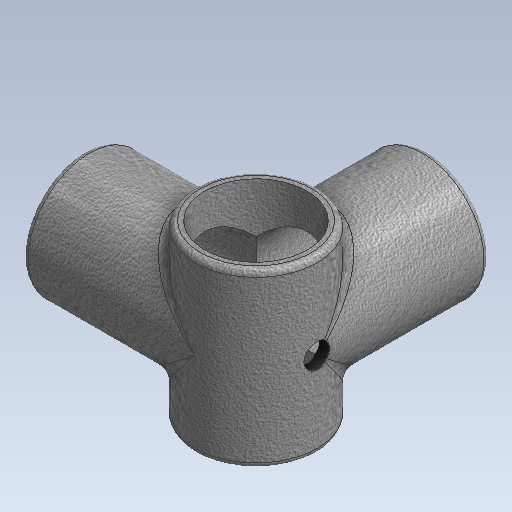
# Autodesk Inventor part: L21-6
Saved by Autodesk Inventor 2021 (Build 250183000, 183)
## iProperties
Created: 2020-04-23
Part Number: L21-6
Material: Aluminium Cast
Document SubType Name: Modeling
Designer: Hannah
Density: 3.00366 g/cm^3
Appearance: Aluminum Cast
Mass: 160 g
Surface Area: 314.88 cm^2
Volume: 53.2684 cm^3
Vendor: Kee Systems
Description: 90 deg side outlet tee
Catalog Web Link: https://keesystems.com/store/fittings/kee-lite/l21-side-outlet-tee.html
Size: 6
Length: n/a
OD: n/a
Author: Hannah
Revision Number: -
Autodesk Inventor part; units mm, degrees
ref_plane "XZ Plane" through (0, 0, 0) normal (0, 1, 0) x (-1, 0, 0)
sketch "Sketch1" plane through (0, 0, 0) normal (0, 0, 1) x (1, 0, 0)
  circle A0 centre (0, 0) radius 17.5
  circle A1 centre (0, 0) radius 21
  dimension "d1" = 42
  dimension "d2" = 35
  constraints: 2 centre point, 2 coincident
  measures "d1" diameter of A1
  measures "d2" diameter of A0
extrude "Extrusion1" add sketch "Sketch1" against normal blind 59 contours A0 | A1
sketch "Sketch2" plane through (0, 0, 0) normal (0, 1, 0) x (-1, 0, 0)
  circle A0 centre (0, 0) radius 17.5
  circle A1 centre (0, 0) radius 21
  dimension "d5" = 35
  dimension "d6" = 42
  constraints: 2 centre point, 2 coincident
  measures "d5" diameter of A0
  measures "d6" diameter of A1
extrude "Extrusion2" add sketch "Sketch2" along normal mid plane 59 contours A0 | A1
ref_plane "Work Plane2" through (0, 0, 0) normal (-0.7071068, 0, 0.7071068) x (0, -1, 0)
mirror "Mirror2" about plane through (0, 0, 0) normal (-0.7071068, 0, 0.7071068) of "Extrusion1"
extrude "Extrusion3" cut sketch "Sketch2" along normal through all both and the other way through all contours A0
extrude "Extrusion4" cut sketch "Sketch1" against normal through all contours A0
mirror "Mirror3" about plane through (0, 0, 0) normal (-0.7071068, 0, 0.7071068) of "Extrusion4"
hole "Hole1" at (0, 0, 0) direction (1, 0, 0) diameter 8.376 end through all thread size "M10x1.5" class "6H" standard "ISO Metric profile"
fillet "Fillet1" radius 5 7 edges at (6.6448, -19.921, -19.921) (6.6448, 19.921, -19.921) (-19.4015, -19.4015, -8.0364) (-14.8492, -14.8492, 14.8492) (-21, 0, -21) (-14.8492, 14.8492, 14.8492) (-19.4015, 19.4015, -8.0364)
fillet "Fillet1" radius 2 4 edges at (21, 29.5, 0) (-59, 0, -21) (-21, 0, -59) (21, -29.5, 0)
sketch "Sketch3" plane through (0, 0, 0) normal (0, 1, 0) x (-1, 0, 0)
  line L0 (-21, -59) -> (21, -59) projected
  line L1 (59, 21) -> (59, -21) projected
  point P0 (0, 0)
  point P1 (44, 0)
  point P2 (0, -44)
  dimension "d43" = 15
  dimension "d44" = 15
  measures "d43" distance from line of L0 point (0, -44)
  measures "d44" distance from line of point (44, 0) L1
hole "Hole3" at (-44, 0, 0) at (0, 0, -44) direction (0, -1, 0) diameter 6.647 end through all thread size "M8x1.25" class "6H" standard "ISO Metric profile"
equation "\"d5\" = d2"
equation "\"d6\" = d1"
body "Solid1"
